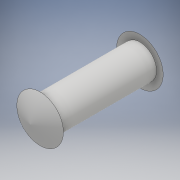
# Autodesk Inventor part: Screw
Saved by Autodesk Inventor 2018 (Build 220112000, 112)
## iProperties
Created: 2019-06-02
Part Number: Screw
Material: Generic
Document SubType Name: Modeling
Designer: dell
Density: 1 g/cm^3
Appearance: Default
Author: dell
Autodesk Inventor part; units mm, degrees
ref_plane "YZ Plane" through (0, 0, 0) normal (1, 0, 0) x (0, 1, 0)
ref_plane "XZ Plane" through (0, 0, 0) normal (0, 1, 0) x (-1, 0, 0)
sketch "Sketch1" plane through (0, 0, 0) normal (0, 1, 0) x (-1, 0, 0)
  circle A0 centre (0, 0) radius 5
  dimension "d0" = 10
  constraints: 1 centre point, 1 coincident
  measures "d0" diameter of A0
extrude "Extrusion1" add sketch "Sketch1" along normal blind 30
sketch "Sketch2" plane through (0, 30, 0) normal (0, 1, 0) x (1, 0, 0)
  point P0 (0, 0)
sketch "Sketch4" plane through (0, 0, 0) normal (0, 0, 1) x (1, 0, 0)
  line L0 (5, 30) -> (-5, 30) projected
  line L1 (0, 30) -> (0, 33)
  arc A0 (7, 30) -> (0, 33) centre (-2.5048, 17.4888) ccw
  line L2 (0, 30) -> (7, 30)
  line L3 (0, -6.6861) -> (0, 40.1166) projected
  point P0 (0, 0)
  dimension "d7" = 3
  dimension "d8" = 7
  constraints: 4 end point, 2 point on circle, 1 centre point, 1 horizontal, 1 midpoint, 1 vertical
  measures "d7" distance of L1.start L1.end
  measures "d8" distance of L1.start L2.end
revolve "Revolution2" add sketch "Sketch4" angle 360 about axis through (0, -10, 0) along (0, 1, 0)
ref_plane "Work Plane2" through (0, 15, 0) normal (0, -1, 0) x (1, 0, 0)
mirror "Mirror2" about plane through (0, 15, 0) normal (0, -1, 0) of "Revolution2"
body "Solid1"
